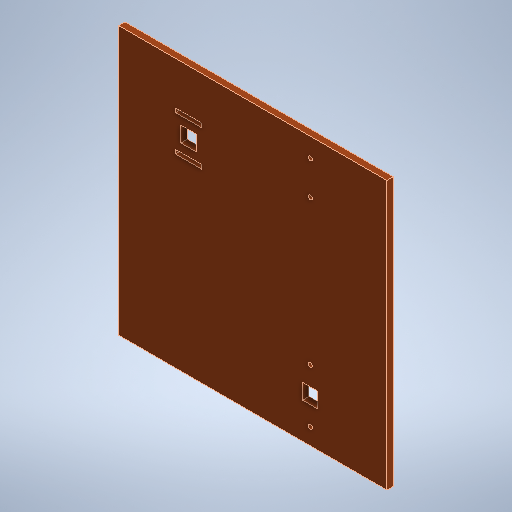
# Autodesk Inventor part: Base
Saved by Autodesk Inventor 2025.4 (Build 294407000, 407)
## iProperties
Created: 2026-04-06
Part Number: Base
Material: Generic
Document SubType Name: Sheet Metal
Designer: lenovo
Density: 1 g/cm^3
Sheet Metal Rule: Default_mm
Appearance: Default(1)
Author: lenovo
Autodesk Inventor part; units mm, degrees
ref_plane "YZ Plane" through (0, 0, 0) normal (1, 0, 0) x (0, 1, 0)
ref_plane "XZ Plane" through (0, 0, 0) normal (0, 1, 0) x (-1, 0, 0)
ref_plane "XY Plane" through (0, 0, 0) normal (0, 0, 1) x (1, 0, 0)
sketch "Sketch1" plane through (0, 0, 0) normal (0, 0, 1) x (1, 0, 0)
  line L0 (-105, -105) -> (105, -105)
  line L1 (105, -105) -> (105, 105)
  line L2 (105, 105) -> (-105, 105)
  line L3 (-105, 105) -> (-105, -105)
  line L4 (-105, -105) -> (105, 105) construction
  line L5 (105, -105) -> (-105, 105) construction
  point P0 (0, 0)
  dimension "d0" = 210
  dimension "d1" = 210
  measures "d0" distance of L1.end L2.end
  measures "d1" distance of L0.end L1.end
extrude "Plate1" add sketch "Sketch1" along normal mid plane 5
sketch "Sketch2" plane through (0, 0, 2.5) normal (0, 0, 1) x (1, 0, 0)
  circle A0 centre (45, 90) radius 1.65
  line L0 (105, 105) -> (105, -105) projected
  line L1 (105, -105) -> (-105, -105) projected
  line L2 (-105, 105) -> (105, 105) projected
  circle A1 centre (45, -92) radius 1.65
  circle A2 centre (45, -50) radius 1.65
  circle A3 centre (45, 63.5) radius 1.65
  point P0 (0, 0)
  dimension "d3" = 3.3
  dimension "d4" = 60
  dimension "d8" = 15
  dimension "d21" = 42
  dimension "d22" = 140
  dimension "d26" = 3.3
  dimension "d27" = 26.5
  constraints: 4 centre point, 3 vertical alignment, 2 equal radius
  measures "d3" diameter of A0
  measures "d4" distance from line of L0 A0.centre
  measures "d8" distance from line of L2 A0.centre
  measures "d21" distance of A2.centre A1.centre
  measures "d22" distance of A2.centre A0.centre
  measures "d26" diameter of A3
  measures "d27" distance of A3.centre A0.centre
extrude "Cut1" cut sketch "Sketch2" against normal blind 5
sketch "Sketch3" plane through (0, 0, 2.5) normal (0, 0, 1) x (1, 0, 0)
  line L0 (-60.5, 71.35) -> (-40, 71.35)
  line L1 (-40, 71.35) -> (-40, 68.25)
  line L2 (-40, 68.25) -> (-60.5, 68.25)
  line L3 (-60.5, 68.25) -> (-60.5, 71.35)
  line L4 (0, 55.75) -> (-105, 55.75)
  line L5 (-105, 105) -> (-105, -105) projected
  line L6 (-50.25, 71.35) -> (-50.25, -105)
  circle A0 centre (45, 90) radius 1.65 projected
  line L7 (105, -105) -> (-105, -105) projected
  line L8 (-60.5, 40.15) -> (-40, 40.15)
  line L9 (-40, 40.15) -> (-40, 43.25)
  line L10 (-40, 43.25) -> (-60.5, 43.25)
  line L11 (-60.5, 43.25) -> (-60.5, 40.15)
  point P0 (0, 0)
  point P1 (-50.25, 40.15)
  dimension "d9" = 3.1
  dimension "d11" = 20.5
  dimension "d12" = 85
  dimension "d14" = 25
  dimension "d15" = 17
  constraints: 20 end point, 5 symmetric about line, 2 horizontal, 2 parallel, 2 point on line, 1 midpoint, 1 perpendicular, 1 vertical, 1 vertical alignment
  measures "d9" distance of L2.end L0.start
  measures "d11" distance of L0.start L0.end
  measures "d12" distance from line of L1 A0.centre
  measures "d14" diameter of L2 L4
  measures "d15" distance edge to line of A0 L0
extrude "Cut2" cut sketch "Sketch3" against normal blind 5 contours L0 L6 L2 L3 | L0 L1 L2 L6 | L10 L9 L8 L6 | L6 L8 L11 L10
sketch "Sketch5" plane through (0, 0, 2.5) normal (0, 0, 1) x (1, 0, 0)
  circle A0 centre (45, -50) radius 1.65 projected
  circle A1 centre (45, -92) radius 1.65 projected
  line L0 (45, -50) -> (45, -92)
  line L1 (39, -65) -> (51, -65)
  line L2 (51, -65) -> (51, -77)
  line L3 (51, -77) -> (39, -77)
  line L4 (39, -77) -> (39, -65)
  line L5 (39, -65) -> (51, -77) construction
  line L6 (51, -65) -> (39, -77) construction
  point P0 (0, 0)
  point P1 (45, -71)
  dimension "d23" = 12
  constraints: 14 end point, 3 midpoint, 2 parallel, 2 perpendicular, 1 horizontal, 1 vertical
  measures "d23" distance of L2.end L3.end
extrude "Cut3" cut sketch "Sketch5" against normal blind 5 contours L1 L2 L3 L0 | L0 L3 L4 L1
sketch "Sketch6" plane through (0, 0, 2.5) normal (0, 0, 1) x (1, 0, 0)
  line L0 (-56.25, 61.75) -> (-44.25, 61.75)
  line L1 (-44.25, 61.75) -> (-44.25, 49.75)
  line L2 (-44.25, 49.75) -> (-56.25, 49.75)
  line L3 (-56.25, 49.75) -> (-56.25, 61.75)
  line L4 (-56.25, 61.75) -> (-44.25, 49.75) construction
  line L5 (-44.25, 61.75) -> (-56.25, 49.75) construction
  line L6 (-60.5, 71.35) -> (-40, 71.35) projected
  line L7 (-40, 68.25) -> (-60.5, 68.25) projected
  point P0 (0, 0)
  point P1 (-50.25, 55.75)
  point P2 (-50.25, 71.35)
  point P3 (-50.25, 68.25)
  dimension "d28" = 12
  dimension "d29" = 12.5
  constraints: 12 end point, 4 midpoint, 2 parallel, 2 perpendicular, 1 horizontal, 1 vertical alignment
  measures "d28" distance of L1.end L2.end
  measures "d29" distance of point (-50.25, 68.25) point (-50.25, 55.75)
extrude "Cut4" cut sketch "Sketch6" against normal blind 5
equation "\"d6\" = Thickness"
equation "\"d17\" = Thickness"
equation "\"d24\" = Thickness"
equation "\"d30\" = Thickness"
equation "\"d2\" = Thickness"
equation "\"BendRadius\" = Thickness"
equation "\"BendReliefWidth\" = Thickness"
equation "\"BendReliefDepth\" = 0.5 * Thickness"
equation "\"TransitionRadius\" = BendRadius"
equation "\"JacobiRadiusSize\" = BendRadius"
equation "\"GapSize\" = Thickness"
equation "\"Thickness\" = 5"
body "Solid1"
